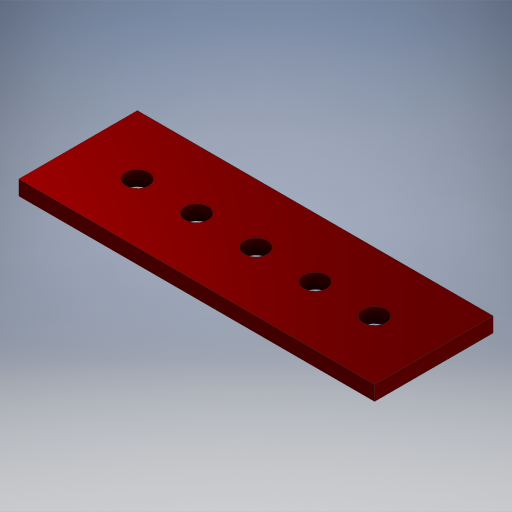
# Autodesk Inventor part: 1x5-Grid-Gusset
Saved by Autodesk Inventor 2024.2 (Build 282272000, 272)
## iProperties
Created: 2024-02-17
Part Number: 1x5-Grid-Gusset
Material: Generic
Document SubType Name: Modeling
Designer: rohan
Density: 1 g/cm^3
Appearance: Default
Author: rohan
Autodesk Inventor part; units mm, degrees
ref_plane "YZ Plane" through (0, 0, 0) normal (1, 0, 0) x (0, 1, 0)
ref_plane "XZ Plane" through (0, 0, 0) normal (0, 1, 0) x (-1, 0, 0)
ref_plane "XY Plane" through (0, 0, 0) normal (0, 0, 1) x (1, 0, 0)
sketch "Sketch1" plane through (0, 0, 0) normal (0, 1, 0) x (-1, 0, 0)
  line L0 (38.1, 12.7) -> (-38.1, 12.7)
  line L1 (-38.1, 12.7) -> (-38.1, -12.7)
  line L2 (-38.1, -12.7) -> (38.1, -12.7)
  line L3 (38.1, -12.7) -> (38.1, 12.7)
  line L4 (38.1, 12.7) -> (-38.1, -12.7) construction
  line L5 (-38.1, 12.7) -> (38.1, -12.7) construction
  circle A0 centre (25.4, 0) radius 2.4892
  circle A1 centre (12.7, 0) radius 2.4892
  circle A2 centre (0, 0) radius 2.4892
  circle A3 centre (-12.7, 0) radius 2.4892
  circle A4 centre (-25.4, 0) radius 2.4892
  point P0 (0, 0)
  point P1 (38.1, 0)
  dimension "d0" = 76.2
  dimension "d1" = 25.4
  dimension "d2" = 4.9784
  dimension "d3" = 12.7
  dimension "d4" = 12.7
  dimension "d7" = 12.7
  dimension "d12" = 12.7
  dimension "d13" = 12.7
  constraints: 12 end point, 5 centre point, 3 midpoint, 2 horizontal, 2 parallel, 1 perpendicular, 8 other
  measures "d0" distance of L2.end L1.end
  measures "d1" distance of L1.end L0.end
  measures "d2" diameter of A0
  measures "d3" distance of point (38.1, 0) A0.centre
  measures "d4" distance from line of L0 A0.centre
  measures "d7" distance of A0.centre A1.centre
  measures "d12" distance from line of L1 A4.centre
  measures "d13" distance from line of L2 A4.centre
extrude "Extrusion1" add sketch "Sketch1" along normal blind 3.175
body "Solid1"
